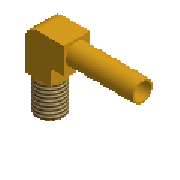
# Autodesk Inventor part: Terminación de manguera para tubería macho 129HB de Parker - Codo de 90° 129HB-4-4
Saved by Autodesk Inventor 2021 (Build 250183000, 183)
## iProperties
NAME: PIPING: Parker Hose Barb 90° Elbow to Male Pipe 129HB
DATA: <meta><inlinegroups number="0" deflen="0"></inlinegroups><connections number="2"></connections><angles><a>1.5707963267949</a></angles></meta>
Created: 2020-01-21
Part Number: Terminación de manguera para tubería macho 129HB de Parker - Codo de 90° 129HB-4-4
Material: Latón, amarillo claro
Description: Terminación de manguera - Codo de 90°
Document SubType Name: Modeling
Standard: Parker
Designer: Admin
Manufacturer: Parker
Language: es-ES
Size Designation: 129HB-4-4
Categories: <MemberInstance><Categories><Category DisplayName="Tubo y tubería" InternalName="4347fa0f-2144-441d-94cd-e3e15c92b736" Mnemonic="TUBEANDPIPE"><CategoryParameter DisplayName="Número de conexiones" InternalName="04e9c83a-9e20-4a98-a7e1-e8abe87a2846" Mnemonic="NUM_CONNECTIONS"/><CategoryParameter DisplayName="Angles" InternalName="0e0e4fa4-3bd3-4656-a22e-4e07c8c476f8" Mnemonic="ANGLES"><CategoryParameter DisplayName="Angle" InternalName="9188ad83-1b16-48b4-8b0a-76ce729dafa7" Mnemonic="ANGLE"/></CategoryParameter><CategoryParameter DisplayName="Clave" InternalName="3da84699-049a-4bc2-a65a-6696b77c242f" Mnemonic="SKEY"/><CategoryParameter DisplayName="Descripción ISOGEN" InternalName="7aa3ba45-b821-4467-8584-f9e6f15f2a7d" Mnemonic="ISOGENDESC"/><CategoryParameter DisplayName="CÓDIGO-ARTÍCULO" InternalName="99cc3b15-24d9-4d38-aac7-792cfbc57acf" Mnemonic="ITEMCODE"/><CategoryParameter DisplayName="NombreDeComponente" InternalName="9c74ad13-48a1-45fe-b0f7-5447561f444a" Mnemonic="NAMEOFCOMPONENT"/><CategoryParameter DisplayName="GruposEnLínea" InternalName="d60be647-bc43-4c18-a13f-9fe4115f8e64" Mnemonic="INLINEGROUPS"/><Category DisplayName="Accesorios" InternalName="ed6b26c4-72b8-4f31-9b63-f85ae8f932e4" Mnemonic="FITTINGS"><CategoryParameter DisplayName="Connections" InternalName="dbd721e8-e885-4eea-9011-b5acfd9f61de" Mnemonic="FIT_CONNECTIONS"><CategoryParameter DisplayName="Tamaño de tubería de conicidencia mín." InternalName="11f51b32-3e37-4310-abf7-f1318a1fd129" Mnemonic="MNMPS"/><CategoryParameter DisplayName="EngraneMáx" InternalName="34fdf028-8797-436e-ba07-ca3dee15bd9b" Mnemonic="MAXENGAGEMENT"/><CategoryParameter DisplayName="TamañoNominal" InternalName="3f94edc7-e459-48db-8f02-8eebf8cffccd" Mnemonic="NS"/><CategoryParameter DisplayName="NombreVisualización" InternalName="50f521dd-e050-43f7-9895-6b30ea7ed42e" Mnemonic="DISPLAYNAME"/><CategoryParameter DisplayName="Cortar tubería de coincidencia" InternalName="53a63a6e-53d8-4ca9-8880-037731d1cceb" Mnemonic="CMP"/><CategoryParameter DisplayName="Género neutro" InternalName="628bd5f1-acad-44e2-9d91-af996ab74fc2" Mnemonic="NEUTRAL"/><CategoryParameter DisplayName="EngraneMín [% de EngraneMáx]" InternalName="7ec1bde5-73f0-45b1-98d8-365a6c67f8ad" Mnemonic="MINENGAGEMENT"/><CategoryParameter DisplayName="Fijo" InternalName="9142902a-6a8a-446d-9eb8-4b7ce7d245ef" Mnemonic="FIXED"/><CategoryParameter DisplayName="Hembra" InternalName="b366bcb5-a500-4bad-84bb-22f956216d69" Mnemonic="FEMALE"/><CategoryParameter DisplayName="DirecciónGiro" InternalName="d55dedc0-f14a-4283-86b4-a4eeb253c8aa" Mnemonic="FLIPDIRECTION"/><CategoryParameter DisplayName="NúmeroPlanificación" InternalName="d6161c62-eb59-4495-a086-874847c10866" Mnemonic="SN"/><CategoryParameter DisplayName="TratamientoFinal" InternalName="d7f11516-3374-45ca-b1c7-4b2d63244ae2" Mnemonic="ENDTREATMENT"/><CategoryParameter DisplayName="Tamaño de tubería de conicidencia máx." InternalName="e73ef66b-c04b-45ac-9b32-f712653e25ee" Mnemonic="MXMPS"/></CategoryParameter><CategoryParameter DisplayName="Connections" InternalName="dbd721e8-e885-4eea-9011-b5acfd9f61de" Mnemonic="FIT_CONNECTIONS"><CategoryParameter DisplayName="Tamaño de tubería de conicidencia mín." InternalName="11f51b32-3e37-4310-abf7-f1318a1fd129" Mnemonic="MNMPS"/><CategoryParameter DisplayName="EngraneMáx" InternalName="34fdf028-8797-436e-ba07-ca3dee15bd9b" Mnemonic="MAXENGAGEMENT"/><CategoryParameter DisplayName="TamañoNominal" InternalName="3f94edc7-e459-48db-8f02-8eebf8cffccd" Mnemonic="NS"/><CategoryParameter DisplayName="NombreVisualización" InternalName="50f521dd-e050-43f7-9895-6b30ea7ed42e" Mnemonic="DISPLAYNAME"/><CategoryParameter DisplayName="Cortar tubería de coincidencia" InternalName="53a63a6e-53d8-4ca9-8880-037731d1cceb" Mnemonic="CMP"/><CategoryParameter DisplayName="Género neutro" InternalName="628bd5f1-acad-44e2-9d91-af996ab74fc2" Mnemonic="NEUTRAL"/><CategoryParameter DisplayName="EngraneMín [% de EngraneMáx]" InternalName="7ec1bde5-73f0-45b1-98d8-365a6c67f8ad" Mnemonic="MINENGAGEMENT"/><CategoryParameter DisplayName="Fijo" InternalName="9142902a-6a8a-446d-9eb8-4b7ce7d245ef" Mnemonic="FIXED"/><CategoryParameter DisplayName="Hembra" InternalName="b366bcb5-a500-4bad-84bb-22f956216d69" Mnemonic="FEMALE"/><CategoryParameter DisplayName="DirecciónGiro" InternalName="d55dedc0-f14a-4283-86b4-a4eeb253c8aa" Mnemonic="FLIPDIRECTION"/><CategoryParameter DisplayName="NúmeroPlanificación" InternalName="d6161c62-eb59-4495-a086-874847c10866" Mnemonic="SN"/><CategoryParameter DisplayName="TratamientoFinal" InternalName="d7f11516-3374-45ca-b1c7-4b2d63244ae2" Mnemonic="ENDTREATMENT"/><CategoryParameter DisplayName="Tamaño de tubería de conicidencia máx." InternalName="e73ef66b-c04b-45ac-9b32-f712653e25ee" Mnemonic="MXMPS"/></CategoryParameter><Category DisplayName="Accesorios de manguera" InternalName="7166b05c-5859-4772-9878-2070c6cbb4c3" Mnemonic="Hose_Fittings"/></Category></Category><Category DisplayName="TipoDatos" InternalName="23b78d0f-2648-40c6-8793-ca6db495c9e8" Mnemonic="DATATYPE"><CategoryParameter DisplayName="NombreVisualización" InternalName="05415f3d-3907-474b-a020-eb9d644f4cf3" Mnemonic="DISPLAYNAME"/><CategoryParameter DisplayName="Estándar" InternalName="0c0a119c-1e12-4c84-803f-101930972f5e" Mnemonic="STANDARD"/><CategoryParameter DisplayName="Descripción" InternalName="13903e3d-64b1-4950-80da-f627842ea37f" Mnemonic="DESCRIPTION"/><CategoryParameter DisplayName="Designación" InternalName="2675968c-4ce5-49e0-a4f5-552d29089031" Mnemonic="DESIGNATION"/><CategoryParameter DisplayName="Fila por defecto" InternalName="2af9ec52-faaa-4026-b378-f9fa4afca842" Mnemonic="DEFAULTROW"/><CategoryParameter DisplayName="Nombre de carpeta" InternalName="3f06958e-8713-4116-9be7-ed6184ecc97b" Mnemonic="FOLDERNAME"/><CategoryParameter DisplayName="Guid de revisión" InternalName="45a75005-10b1-4dfc-8d6d-dfe629f0b93c" Mnemonic="REVISIONGUID"/><CategoryParameter DisplayName="NombreArchivo" InternalName="8b46a4cc-9585-4fed-90c3-899f57e09a73" Mnemonic="FILENAME"/><CategoryParameter DisplayName="OrgEstand" InternalName="8f5914e1-4693-403f-8ab5-d37768198c9d" Mnemonic="STDSORG"/><CategoryParameter DisplayName="Versión de familia" InternalName="914462f6-6e19-4b14-ba84-155b9680b1d0" Mnemonic="FAMILYREVISION"/><CategoryParameter DisplayName="Revisión de Norma" InternalName="91d5a463-65c2-4fde-b823-3b7fea5e8e17" Mnemonic="STANDARDREVISION"/><CategoryParameter DisplayName="Revisión del miembro" InternalName="a65d44b9-392f-4f4f-857b-e4b3d54996fe" Mnemonic="MEMBERREVISION"/><CategoryParameter DisplayName="FormatoDelimitación" InternalName="bc51e27b-3422-4e78-93ef-cec197ddf230" Mnemonic="CLIPFORMAT"/><CategoryParameter DisplayName="Fabricante" InternalName="cd6c7a72-a28a-4e50-99a9-2c7f4e13e5ad" Mnemonic="MANUFACTURER"/><CategoryParameter DisplayName="NombreInterno" InternalName="cf1d0246-76d9-4b4a-8305-fa0409afb5c1" Mnemonic="INTERNALNAME"/><CategoryParameter DisplayName="EsMétrico" InternalName="e2385c5b-1ea4-4823-96a8-8de651266ec3" Mnemonic="ISMETRIC"/><Category DisplayName="Pieza" InternalName="c0e0b642-3bcb-4cc8-9e80-f96d35c4afa4" Mnemonic="PART"><CategoryParameter DisplayName="Número de pieza" InternalName="016b6077-bfbe-49bd-92c9-d8d59c39c941" Mnemonic="PARTNUMBER"/><CategoryParameter DisplayName="Referencia de almacén" InternalName="4dba7c1c-e26c-444e-836c-b08b433409a8" Mnemonic="STOCKNUMBER"/><CategoryParameter DisplayName="Clave de material" InternalName="5c9a8adb-dd2b-4535-b97f-0a94a95fe41f" Mnemonic="MATERIALKEY"/><CategoryParameter DisplayName="Material" InternalName="818a152a-d3c3-49ca-80ee-df7d91421b8e" Mnemonic="MATERIAL"/></Category></Category><Category DisplayName="AsignaciónHeredada" InternalName="dfeab48a-acc2-4514-a11c-1b8dc28c3d5f" Mnemonic="LEGACYMAP"><CategoryParameter DisplayName="IDCatálogo" InternalName="0da51c36-8fd3-4028-86cc-0c9c9e96136a" Mnemonic="CATALOGID"/><CategoryParameter DisplayName="IDFamilia" InternalName="1c0b589c-8bbe-4e1e-80cf-07c0de42ac2a" Mnemonic="FAMILYID"/><CategoryParameter DisplayName="IDMiembro" InternalName="a368ea03-db8a-4d6e-962b-2aa46306b8f5" Mnemonic="MEMBERID"/></Category></Categories><FamilyTemplate Id="Parker Hose Barb 90° Elbow to Male Pipe 129HB"><FamilyTemplateParameters><FamilyTemplateParameter ObjectType="kUserParameterObject" ValueType="xs:double" Id="1" ObjectReferenceKey="L1"/><FamilyTemplateParameter ObjectType="kUserParameterObject" ValueType="xs:double" Id="2" ObjectReferenceKey="M1"/><FamilyTemplateParameter ObjectType="kUserParameterObject" ValueType="xs:double" Id="3" ObjectReferenceKey="N1"/><FamilyTemplateParameter ObjectType="kUserParameterObject" ValueType="xs:double" Id="4" ObjectReferenceKey="OD"/><FamilyTemplateParameter ObjectType="kUserParameterObject" ValueType="xs:double" Id="5" ObjectReferenceKey="D1"/><FamilyTemplateParameter ObjectType="kUserParameterObject" ValueType="xs:double" Id="6" ObjectReferenceKey="DT"/><FamilyTemplateParameter ObjectType="kUserParameterObject" ValueType="xs:string" Id="119" ObjectReferenceKey="Parker_No"/><FamilyTemplateParameter ObjectType="kPropertyObject" ValueType="xs:string" Id="100" ObjectReferenceKey="{32853F0F-3444-11d1-9E93-0060B03C1CA6}" SubObjectId="52"/><FamilyTemplateParameter ObjectType="kPropertyObject" ValueType="xs:string" Id="105" ObjectReferenceKey="{32853F0F-3444-11d1-9E93-0060B03C1CA6}" SubObjectId="5"/><FamilyTemplateParameter ObjectType="kPartComponentDefinitionObject" ValueType="xs:string" Id="110" SubObjectId="Material"/><FamilyTemplateParameter ObjectType="kThreadFeatureObject" ValueType="xs:structure" Id="300" ObjectReferenceKey="10020000100000008C600000000000008000000000000000" SubObjectId="ThreadInfo"><FamilyTemplateParameter ObjectType="" ValueType="xs:string" Id="301" SubObjectId="ThreadType"/><FamilyTemplateParameter ObjectType="" ValueType="xs:string" Id="302" SubObjectId="NominalDiameter"/></FamilyTemplateParameter></FamilyTemplateParameters></FamilyTemplate><CategoryParameterMap><ParamToTemplateMap><ParamToTemplate CategoryParameter="//CategoryParameter[@InternalName='d60be647-bc43-4c18-a13f-9fe4115f8e64']" ConstantValue="0"/><ParamToTemplate CategoryParameter="//CategoryParameter[@InternalName='04e9c83a-9e20-4a98-a7e1-e8abe87a2846']" ConstantValue="2"/><ParamToTemplate CategoryParameter="//CategoryParameter[@InternalName='0e0e4fa4-3bd3-4656-a22e-4e07c8c476f8']" ConstantValue=""/><ParamToTemplate CategoryParameter="//CategoryParameter[@InternalName='0e0e4fa4-3bd3-4656-a22e-4e07c8c476f8'][1]/CategoryParameter[@InternalName='9188ad83-1b16-48b4-8b0a-76ce729dafa7']" ConstantValue="1.5707963267949"/><ParamToTemplate CategoryParameter="//CategoryParameter[@InternalName='9c74ad13-48a1-45fe-b0f7-5447561f444a']" ConstantValue="ELBOW"/><ParamToTemplate CategoryParameter="//CategoryParameter[@InternalName='dbd721e8-e885-4eea-9011-b5acfd9f61de'][1]/CategoryParameter[@InternalName='d55dedc0-f14a-4283-86b4-a4eeb253c8aa']" ConstantValue="false"/><ParamToTemplate CategoryParameter="//CategoryParameter[@InternalName='dbd721e8-e885-4eea-9011-b5acfd9f61de'][1]/CategoryParameter[@InternalName='50f521dd-e050-43f7-9895-6b30ea7ed42e']" ConstantValue="Connection1"/><ParamToTemplate CategoryParameter="//CategoryParameter[@InternalName='dbd721e8-e885-4eea-9011-b5acfd9f61de'][1]/CategoryParameter[@InternalName='b366bcb5-a500-4bad-84bb-22f956216d69']" ConstantValue="false"/><ParamToTemplate CategoryParameter="//CategoryParameter[@InternalName='dbd721e8-e885-4eea-9011-b5acfd9f61de'][1]/CategoryParameter[@InternalName='d7f11516-3374-45ca-b1c7-4b2d63244ae2']" ConstantValue="Quick Connection"/><ParamToTemplate CategoryParameter="//CategoryParameter[@InternalName='dbd721e8-e885-4eea-9011-b5acfd9f61de'][1]/CategoryParameter[@InternalName='9142902a-6a8a-446d-9eb8-4b7ce7d245ef']" ConstantValue="false"/><ParamToTemplate CategoryParameter="//CategoryParameter[@InternalName='dbd721e8-e885-4eea-9011-b5acfd9f61de'][1]/CategoryParameter[@InternalName='34fdf028-8797-436e-ba07-ca3dee15bd9b']" ConstantValue="0"/><ParamToTemplate CategoryParameter="//CategoryParameter[@InternalName='dbd721e8-e885-4eea-9011-b5acfd9f61de'][1]/CategoryParameter[@InternalName='7ec1bde5-73f0-45b1-98d8-365a6c67f8ad']" ConstantValue="50"/><ParamToTemplate CategoryParameter="//CategoryParameter[@InternalName='dbd721e8-e885-4eea-9011-b5acfd9f61de'][2]/CategoryParameter[@InternalName='d55dedc0-f14a-4283-86b4-a4eeb253c8aa']" ConstantValue="false"/><ParamToTemplate CategoryParameter="//CategoryParameter[@InternalName='dbd721e8-e885-4eea-9011-b5acfd9f61de'][2]/CategoryParameter[@InternalName='50f521dd-e050-43f7-9895-6b30ea7ed42e']" ConstantValue="Connection2"/><ParamToTemplate CategoryParameter="//CategoryParameter[@InternalName='dbd721e8-e885-4eea-9011-b5acfd9f61de'][2]/CategoryParameter[@InternalName='b366bcb5-a500-4bad-84bb-22f956216d69']" ConstantValue="false"/><ParamToTemplate CategoryParameter="//CategoryParameter[@InternalName='dbd721e8-e885-4eea-9011-b5acfd9f61de'][2]/CategoryParameter[@InternalName='d7f11516-3374-45ca-b1c7-4b2d63244ae2']" ConstantValue="Threaded"/><ParamToTemplate CategoryParameter="//CategoryParameter[@InternalName='dbd721e8-e885-4eea-9011-b5acfd9f61de'][2]/CategoryParameter[@InternalName='9142902a-6a8a-446d-9eb8-4b7ce7d245ef']" ConstantValue="false"/><ParamToTemplate CategoryParameter="//CategoryParameter[@InternalName='dbd721e8-e885-4eea-9011-b5acfd9f61de'][2]/CategoryParameter[@InternalName='34fdf028-8797-436e-ba07-ca3dee15bd9b']" ConstantValue="0"/><ParamToTemplate CategoryParameter="//CategoryParameter[@InternalName='dbd721e8-e885-4eea-9011-b5acfd9f61de'][2]/CategoryParameter[@InternalName='7ec1bde5-73f0-45b1-98d8-365a6c67f8ad']" ConstantValue="50"/><ParamToTemplate CategoryParameter="//CategoryParameter[@InternalName='05415f3d-3907-474b-a020-eb9d644f4cf3']" ConstantValue="Parker Hose Barb 90° Elbow to Male Pipe 129HB"/><ParamToTemplate CategoryParameter="//CategoryParameter[@InternalName='cf1d0246-76d9-4b4a-8305-fa0409afb5c1']" ConstantValue="7ab0a660-a435-4c12-aa15-99a8a8310ea8"/><ParamToTemplate CategoryParameter="//CategoryParameter[@InternalName='3f06958e-8713-4116-9be7-ed6184ecc97b']" ConstantValue="Parker Hose Barb 90deg Elbow to Male Pipe 129HB"/><ParamToTemplate CategoryParameter="//CategoryParameter[@InternalName='914462f6-6e19-4b14-ba84-155b9680b1d0']" ConstantValue="10"/><ParamToTemplate CategoryParameter="//CategoryParameter[@InternalName='13903e3d-64b1-4950-80da-f627842ea37f']" ConstantValue="Hose Barb 90° Elbow"/><ParamToTemplate CategoryParameter="//CategoryParameter[@InternalName='8f5914e1-4693-403f-8ab5-d37768198c9d']" TemplateParameter="101"/><ParamToTemplate CategoryParameter="//CategoryParameter[@InternalName='0c0a119c-1e12-4c84-803f-101930972f5e']" ConstantValue="Parker"/><ParamToTemplate CategoryParameter="//CategoryParameter[@InternalName='cd6c7a72-a28a-4e50-99a9-2c7f4e13e5ad']" ConstantValue="Parker"/><ParamToTemplate CategoryParameter="//CategoryParameter[@InternalName='91d5a463-65c2-4fde-b823-3b7fea5e8e17']" TemplateParameter="103"/><ParamToTemplate CategoryParameter="//CategoryParameter[@InternalName='bc51e27b-3422-4e78-93ef-cec197ddf230']" ConstantValue="CF_INVENTOR.STDPARTS"/><ParamToTemplate CategoryParameter="//CategoryParameter[@InternalName='e2385c5b-1ea4-4823-96a8-8de651266ec3']" ConstantValue="false"/><ParamToTemplate CategoryParameter="//CategoryParameter[@InternalName='45a75005-10b1-4dfc-8d6d-dfe629f0b93c']" ConstantValue="033f723a-b253-4858-993a-658cf7c5185e"/><ParamToTemplate CategoryParameter="//CategoryParameter[@InternalName='2af9ec52-faaa-4026-b378-f9fa4afca842']" ConstantValue="1"/><ParamToTemplate CategoryParameter="//CategoryParameter[@InternalName='0da51c36-8fd3-4028-86cc-0c9c9e96136a']" ConstantValue="FD8AAA93-B897-476C-BD5D-67C712EC5ABF"/><ParamToTemplate CategoryParameter="//CategoryParameter[@InternalName='1c0b589c-8bbe-4e1e-80cf-07c0de42ac2a']" ConstantValue="7ab0a660-a435-4c12-aa15-99a8a8310ea8"/><ParamToTemplate CategoryParameter="//CategoryParameter[@InternalName='99cc3b15-24d9-4d38-aac7-792cfbc57acf']" ConstantValue=""/><ParamToTemplate CategoryParameter="//CategoryParameter[@InternalName='7aa3ba45-b821-4467-8584-f9e6f15f2a7d']" ConstantValue=""/><ParamToTemplate CategoryParameter="//CategoryParameter[@InternalName='dbd721e8-e885-4eea-9011-b5acfd9f61de'][1]/CategoryParameter[@InternalName='3f94edc7-e459-48db-8f02-8eebf8cffccd']" ConstantValue="1/4"/><ParamToTemplate CategoryParameter="//CategoryParameter[@InternalName='dbd721e8-e885-4eea-9011-b5acfd9f61de'][2]/CategoryParameter[@InternalName='3f94edc7-e459-48db-8f02-8eebf8cffccd']" ConstantValue="1/4"/><ParamToTemplate CategoryParameter="//CategoryParameter[@InternalName='8b46a4cc-9585-4fed-90c3-899f57e09a73']" ConstantValue="Parker Hose Barb 90° Elbow to Male Pipe 129HB 129HB-4-4"/><ParamToTemplate CategoryParameter="//CategoryParameter[@InternalName='a65d44b9-392f-4f4f-857b-e4b3d54996fe']" ConstantValue="b18b5294-f9be-48da-8bc9-0e234296c71f"/><ParamToTemplate CategoryParameter="//CategoryParameter[@InternalName='a368ea03-db8a-4d6e-962b-2aa46306b8f5']" ConstantValue="AEAC944C-49EA-4417-830E-2A202B33B226"/><ParamToTemplate CategoryParameter="//CategoryParameter[@InternalName='2675968c-4ce5-49e0-a4f5-552d29089031']" TemplateParameter="100"/><ParamToTemplate CategoryParameter="//CategoryParameter[@InternalName='818a152a-d3c3-49ca-80ee-df7d91421b8e']" TemplateParameter="110"/><ParamToTemplate CategoryParameter="//CategoryParameter[@InternalName='016b6077-bfbe-49bd-92c9-d8d59c39c941']" TemplateParameter="105"/></ParamToTemplateMap></CategoryParameterMap></MemberInstance>
Density: 8.47 g/cm^3
Appearance: Latón - Satinado
IsCustomPart: 0
Author: Admin
Autodesk Inventor part; units mm, degrees
ref_plane "YZ Plane" through (0, 0, 0) normal (1, 0, 0) x (0, 1, 0)
ref_plane "XZ Plane" through (0, 0, 0) normal (0, 1, 0) x (-1, 0, 0)
ref_plane "XY Plane" through (0, 0, 0) normal (0, 0, 1) x (1, 0, 0)
sketch "Sketch2" plane through (0, 0, 0) normal (0, 1, 0) x (-1, 0, 0)
  circle A0 centre (0, 0) radius 6.0629
  dimension "d0" = 12.1257
  constraints: 1 centre point, 1 coincident, 2 other
  measures "d0" diameter of A0
extrude "Extrusion1" add sketch "Sketch2" along normal blind 10.922 draft 1.79
chamfer "Chamfer1" distance 0.3683 angle 45 1 edges at (6.0629, 0, 0)
sketch "Sketch13" plane through (0, 0, 0) normal (0, 0, 1) x (1, 0, 0)
  line L0 (0, 0) -> (0, 49.334)
  line L1 (26.924, 21.844) -> (26.924, 24.6939)
  line L2 (15.685, 0) -> (0, 0)
  line L3 (26.924, 24.6939) -> (22.098, 25.527)
  line L4 (22.098, 25.527) -> (22.098, 24.6939)
  line L5 (22.098, 24.6939) -> (17.272, 25.527)
  line L6 (17.272, 25.527) -> (17.272, 24.6939)
  line L7 (17.272, 24.6939) -> (12.446, 25.527)
  line L8 (12.446, 25.527) -> (12.446, 24.6939)
  line L9 (12.446, 24.6939) -> (7.62, 25.527)
  line L10 (7.62, 25.527) -> (7.62, 26.2636)
  line L11 (7.62, 26.2636) -> (0, 26.2636)
  line L12 (-10.1194, 21.844) -> (26.924, 21.844)
  line L13 (0, 21.844) -> (0, 26.2636)
  dimension "d57" = 26.924
  dimension "d60" = 4.826
  dimension "d61" = 4.826
  dimension "d62" = 4.826
  dimension "d79" = 19.304
  dimension "d80" = 21.844
  dimension "d81" = 8.8392
  dimension "d84" = 7.366
  dimension "d85" = 5.6998
  constraints: 28 end point, 7 parallel, 4 horizontal alignment, 3 perpendicular, 2 point on line, 1 coincident, 1 horizontal
  measures "d57" distance between parallel lines of L1 L0
  measures "d60" distance between parallel lines of L1 L4
  measures "d61" distance between parallel lines of L6 L4
  measures "d62" distance between parallel lines of L8 L6
  measures "d79" distance between parallel lines of L1 L10
  measures "d80" distance between parallel lines of L2 L12
  measures "d81" diameter of L11 L12
  measures "d84" diameter of L3.end L12
  measures "d85" diameter of L1.end L12
revolve "Revolution3" add sketch "Sketch13" angle 360 about axis through (-10.1194, 21.844, 0) along (1, 0, 0)
ref_plane "Work Plane3" through (0, 11.7958, 0) normal (0, 1, 0) x (1, 0, 0)
sketch "Sketch15" plane through (0, 11.7958, 0) normal (0, 1, 0) x (1, 0, 0)
  circle A0 centre (0, 0) radius 6.4042 projected
  circle A1 centre (0.1637, 0) radius 6.2405
  line L0 (-6.0768, -6.2405) -> (-6.0768, 6.2405)
  line L1 (6.4042, 6.2405) -> (-6.0768, 6.2405)
  line L2 (6.4042, 0) -> (6.4042, 6.2405)
  line L3 (6.4042, 0) -> (6.4042, -6.2405)
  line L4 (6.4042, -6.2405) -> (-6.0768, -6.2405)
  dimension "d71" = 0.1637
  dimension "d104" = 0
  constraints: 10 end point, 5 vertical, 2 horizontal, 2 horizontal alignment, 2 perpendicular, 1 collinear, 3 other
  measures "d71" distance of point (0.164, 0) point (0, 0)
  measures "d104" vertical distance of point (0, 0) point (0.164, 0)
extrude "Extrusion5" add sketch "Sketch15" along normal blind 7.8638 contours A1
loft "Loft2" add section 1 edges at (6.4042, 10.922, 0) section 2 edges at (-6.0768, 11.7958, 0)
ref_plane "Work Plane4" through (-6.0768, 11.7958, 0) normal (1, 0, 0) x (0, 1, 0)
sketch "Sketch22" plane through (7.62, 21.844, 0) normal (1, 0, 0) x (0, 0, -1)
  line L0 (-6.2405, 4.4196) -> (6.2405, 4.4196)
  line L1 (6.2405, 4.4196) -> (6.2405, -4.4196)
  line L2 (6.2405, -4.4196) -> (-6.2405, -4.4196)
  line L3 (-6.2405, -4.4196) -> (-6.2405, 4.4196)
  line L4 (-6.2405, -10.0482) -> (-6.2405, -2.1844) projected
  line L5 (6.2405, -10.0482) -> (6.2405, -2.1844) projected
  circle A0 centre (0, 0) radius 4.4196 projected
  constraints: 8 end point, 2 parallel, 2 point on line, 2 tangent, 1 horizontal, 1 perpendicular
extrude "Extrusion8" add sketch "Sketch22" against normal up to surface (13.6968 mm away)
sketch "Sketch26" plane through (-6.0768, 17.4244, 6.2405) normal (0, -1, 0) x (1, 0, 0)
  arc A0 (6.2405, 0) -> (0, -6.2405) centre (6.2405, -6.2405) ccw projected
  arc A1 (6.2405, 0) -> (0, -6.2405) centre (6.2405, -6.2405) ccw projected
  line L0 (6.2405, 0) -> (0, 0) projected
  line L1 (0, -6.2405) -> (0, 0) projected
  arc A2 (0, -6.2405) -> (6.2405, -12.481) centre (6.2405, -6.2405) ccw projected
  line L2 (0, -12.481) -> (0, -6.2405) projected
  line L3 (6.2405, -12.481) -> (0, -12.481) projected
extrude "Extrusion11" cut sketch "Sketch26" against normal up to next
sketch "Sketch27" plane through (7.62, 17.4244, 6.2405) normal (0, 0, 1) x (1, 0, 0)
  arc A0 (-7.4563, 8.8392) -> (-13.6968, 2.5987) centre (-7.4563, 2.5987) ccw
  line L0 (0, 8.8392) -> (-7.4563, 8.8392) projected
  line L1 (-13.6968, -5.6286) -> (-13.6968, 8.8392) projected
  line L2 (-7.4563, 8.8392) -> (-13.6968, 8.8392) projected
  constraints: 2 point on circle, 2 tangent, 1 centre point, 1 point on line
extrude "Extrusion12" cut sketch "Sketch27" against normal up to next
thread "Rosca2" size "1/4" designation "1/4 - 18 NPT" standard "NPT for PVC Pipe and Fitting" full length
sketch "Sketch28" plane through (7.62, 17.4244, 6.2405) normal (0, 0, 1) x (1, 0, 0)
  line L0 (0, 8.8392) -> (-7.4563, 8.8392) projected
  line L1 (-1.2158, -5.6286) -> (-1.2158, 0) projected
  line L2 (-13.6968, -5.6286) -> (-1.2158, -5.6286) projected
  line L3 (-13.6968, -5.6286) -> (-13.6968, 2.5987) projected
  line L4 (-1.2158, -5.6286) -> (-13.6968, -5.6286)
  line L5 (-13.6968, -5.6286) -> (-13.6968, 8.8392)
  line L6 (-13.6968, 8.8392) -> (-1.2158, 8.8392)
  line L7 (-1.2158, 8.8392) -> (-1.2158, -5.6286)
  constraints: 8 end point, 2 collinear, 2 parallel, 1 horizontal, 1 perpendicular
extrude "Extrusion13" add sketch "Sketch28" against normal up to surface (12.481 mm away)
hole "Hole1" at (26.924, 21.844, 0) direction (-1, 0, 0) diameter 4.7498 depth 26.924 tip angle 118
hole "Hole2" at (0, 0, 0) direction (0, 1, 0) diameter 4.7498 depth 21.844 tip angle 118 countersink diameter 5.6998 countersink angle 82
fillet "Fillet4" radius 4.3688 1 edges at (-6.0768, 26.2636, 0)
fillet "Fillet5" radius 1.0922 1 edges at (6.4042, 17.4244, 0)
equation "\"d0\" = DT"
equation "\"d1\" = 0.5 * N1"
equation "\"d3\" = 0.05 * OD"
equation "\"d57\" = L1"
equation "\"d60\" = 0.25 * M1"
equation "\"d61\" = 0.25 * M1"
equation "\"d62\" = 0.25 * M1"
equation "\"d79\" = M1"
equation "\"d80\" = N1"
equation "\"d81\" = 1.2 * OD"
equation "\"d84\" = OD"
equation "\"d85\" = 1.2 * D1"
equation "\"d71\" = 0.0222222 * OD"
equation "\"d73\" = 0.36 * N1"
equation "\"d111\" = D1"
equation "\"d120\" = D1"
equation "\"d122\" = 1.2 * D1"
equation "\"d125\" = N1"
equation "\"d129\" = 0.2 * N1"
equation "\"d130\" = 0.05 * N1"
equation "\"L1\" = 26.924"
equation "\"M1\" = 19.304"
equation "\"N1\" = 21.844"
equation "\"OD\" = 7.366"
equation "\"D1\" = 4.7498"
equation "\"d70\" = 0.04 * N1"
equation "\"DT\" = 12.12571"
equation "\"Parker_No\" = 1.2345"
body "Solid1"
